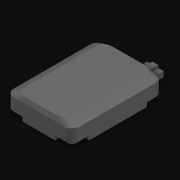
# Autodesk Inventor part: V5 Simple Brain
Saved by Autodesk Inventor 2025.2 (Build 292293000, 293)
## iProperties
Created: 2020-06-02
Part Number: V5 Simple Brain
Material: Generic
Document SubType Name: Modeling
Designer: yuany
Density: 1 g/cm^3
Appearance: Default
Author: yuany
Autodesk Inventor part; units mm, degrees
ref_plane "YZ Plane" through (0, 0, 0) normal (1, 0, 0) x (0, 1, 0)
ref_plane "XZ Plane" through (0, 0, 0) normal (0, 1, 0) x (-1, 0, 0)
ref_plane "XY Plane" through (0, 0, 0) normal (0, 0, 1) x (1, 0, 0)
sketch "Sketch1" plane through (0, 0, 0) normal (0, 1, 0) x (-1, 0, 0)
  line L0 (-49.911, 68.961) -> (49.911, 68.961)
  line L1 (49.911, 68.961) -> (49.911, -68.961)
  line L2 (49.911, -68.961) -> (-49.911, -68.961)
  line L3 (-49.911, -68.961) -> (-49.911, 68.961)
  point P0 (0, 0)
  dimension "d0" = 137.922
  dimension "d1" = 99.822
  dimension "d66" = 49.911
  dimension "d67" = 68.961
  constraints: 8 end point, 2 parallel, 1 horizontal, 1 perpendicular
  measures "d0" distance of L0.end L1.end
  measures "d1" distance of L1.end L2.end
  measures "d66" distance from line of point (0, 0) L1
  measures "d67" distance from line of point (0, 0) L0
extrude "Extrusion1" add sketch "Sketch1" along normal mid plane 31.4706
chamfer "Chamfer2" distance 2.921 distance2 6.35 1 edges at (0, 15.7353, 68.961) measured on face at (0, 15.7353, 68.461)
chamfer "Chamfer3" distance 2.921 distance2 6.35 1 edges at (0, 15.7353, -68.961) measured on face at (0, 15.7353, -68.461)
chamfer "Chamfer4" distance 12.7 distance2 6.35 1 edges at (49.911, 15.7353, 0) measured on face at (49.411, 15.7353, 0)
chamfer "Chamfer5" distance 12.7 distance2 6.35 1 edges at (-49.911, 15.7353, 0) measured on face at (-49.411, 15.7353, 0)
fillet "Fillet5" radius 11.811 8 edges at (-49.911, -3.175, -68.961) (-49.911, -3.175, 68.961) (49.911, -3.175, -68.961) (-43.561, 12.5603, -67.5005) (-43.561, 12.5603, 67.5005) (43.561, 12.5603, 67.5005) (43.561, 12.5603, -67.5005) (49.911, -3.175, 68.961)
fillet "Fillet6" radius 6.35 7 edges at (-46.4516, -15.7353, 65.5016) (0, -15.7353, 68.961) (49.911, -15.7353, 0) (46.4516, -15.7353, -65.5016) (0, -15.7353, -68.961) (-46.4516, -15.7353, -65.5016) (-49.911, -15.7353, 0) inverted yes
sketch "Sketch4" plane through (-49.911, 9.3853, -57.15) normal (-1, 0, 0) x (0, 0, 1)
  line L0 (114.3, -25.1206) -> (0, -25.1206) projected
  line L1 (12.7, -16.8159) -> (101.6, -16.8159)
  line L2 (101.6, -16.8159) -> (101.6, -25.1206)
  line L3 (101.6, -25.1206) -> (12.7, -25.1206)
  line L4 (12.7, -25.1206) -> (12.7, -16.8159)
  line L5 (0, 0) -> (114.3, 0) projected
  point P0 (57.15, -9.3853)
  point P1 (12.7, -25.1206)
  point P2 (119.761, -25.1206)
  dimension "d34" = 88.9
  dimension "d35" = 12.7
  constraints: 8 end point, 2 parallel, 1 horizontal, 1 perpendicular, 1 point on line
  measures "d34" distance of L2.end L3.end
  measures "d35" distance from line of L5.start L4
extrude "Extrusion4" add sketch "Sketch4" against normal up to surface (99.822 mm away)
sketch "Sketch5" plane through (-33.3726, 9.3853, 68.961) normal (0, 0, 1) x (1, 0, 0)
  line L0 (7.9756, -14.607) -> (58.7756, -14.607)
  line L1 (58.7756, -14.607) -> (58.7756, -25.1206)
  line L2 (58.7756, -25.1206) -> (7.9756, -25.1206)
  line L3 (7.9756, -25.1206) -> (7.9756, -14.607)
  line L4 (0, 0) -> (66.7451, 0) projected
  point P0 (33.3726, -9.3853)
  dimension "d38" = 50.8
  dimension "d39" = 7.9756
  constraints: 8 end point, 2 parallel, 1 horizontal, 1 perpendicular
  measures "d38" distance of L1.end L2.end
  measures "d39" distance from line of L4.start L3
extrude "Extrusion5" add sketch "Sketch5" against normal up to surface (137.922 mm away)
fillet "Fillet7" radius 2.0066 8 edges at (25.403, -15.7353, 65.786) (46.736, -15.7353, 44.45) (-25.397, -15.7353, 65.786) (-46.736, -15.7353, 44.45) (-46.736, -15.7353, -44.45) (-25.397, -15.7353, -65.786) (46.736, -15.7353, -44.45) (25.403, -15.7353, -65.786)
fillet "Fillet8" radius 0.254 47 edges at (43.5812, -15.2289, -43.776) (46.1975, -10.5844, -44.45) (46.4516, -9.3853, -65.5016) (31.7515, -9.3853, -68.961) (49.911, -9.3853, -50.8) (49.911, -15.1476, -43.8623) (49.911, -15.7353, 0) (49.911, -15.1476, 43.8623) (49.911, -11.557, 44.45) (49.911, -11.557, -44.45) (24.729, -15.2289, -62.6312) (25.403, -10.5844, -65.2475) (24.8153, -15.1476, -68.961) (0.003, -15.7353, -68.961) (-24.8092, -15.1476, -68.961) (-25.397, -11.557, -68.961) (25.403, -11.557, -68.961) (24.7268, -15.2309, 62.6311) (25.403, -10.5844, 65.2475) (49.911, -9.3853, 50.8) (31.7515, -9.3853, 68.961) (-31.7485, -9.3853, 68.961) (24.8153, -15.1476, 68.961) (0.003, -15.7353, 68.961) (-24.8092, -15.1476, 68.961) (-25.397, -11.557, 68.961) (25.403, -11.557, 68.961) (43.5812, -15.2289, 43.776) (46.1975, -10.5844, 44.45) (-43.5812, -15.2289, 43.776) (-46.1975, -10.5844, 44.45) (-46.4516, -9.3853, 65.5016) (-49.911, -9.3853, 50.8) (-24.723, -15.2289, 62.6312) (-25.397, -10.5844, 65.2475) (-49.911, -15.1476, 43.8623) (-49.911, -11.557, 44.45) (-49.911, -15.1476, -43.8623) (-49.911, -11.557, -44.45) (-49.911, -15.7353, 0) (-24.723, -15.2289, -62.6312) (-25.397, -10.5844, -65.2475) (-43.5812, -15.2289, -43.776) (-46.1975, -10.5844, -44.45) (-46.4516, -9.3853, -65.5016) (-31.7485, -9.3853, -68.961) (-49.911, -9.3853, -50.8)
sketch "Sketch6" plane through (0, -15.7353, 0) normal (0, -1, 0) x (1, 0, 0)
  circle A0 centre (19.053, 38.1) radius 1.7272
  line L0 (49.657, 42.4434) -> (49.657, -42.4434) projected
  line L1 (-23.3904, 68.707) -> (23.3964, 68.707) projected
  circle A1 centre (19.053, -38.1) radius 1.7272
  circle A2 centre (-19.047, 38.1) radius 1.7272
  circle A3 centre (-19.047, -38.1) radius 1.7272
  point P0 (0, 0)
  dimension "d44" = 3.4544
  dimension "d47" = 76.2
  dimension "d50" = 38.1
  dimension "d53" = 4.3434
  dimension "d54" = 4.3434
  constraints: 4 centre point, 1 horizontal, 1 vertical, 6 other
  measures "d44" diameter of A0
  measures "d47" distance of A0.centre A1.centre
  measures "d50" distance of A0.centre A2.centre
  measures "d53" vertical distance of A0.centre L0.start
  measures "d54" horizontal distance of A0.centre L1.end
extrude "Extrusion6" cut sketch "Sketch6" against normal blind 6.35
sketch "Sketch7" plane through (33.3726, 9.3853, -68.961) normal (0, 0, -1) x (-1, 0, 0)
  line L0 (-0.9809, -5.8547) -> (23.7079, -5.8547)
  line L1 (23.7079, -5.8547) -> (23.7079, -14.0843)
  line L2 (23.7079, -14.0843) -> (-0.9809, -14.0843)
  line L3 (-0.9809, -14.0843) -> (-0.9809, -5.8547)
  line L4 (6.9693, -5.8547) -> (15.8085, -5.8547)
  line L5 (15.8085, -5.8547) -> (15.8085, -1.9685)
  line L6 (15.8085, -1.9685) -> (6.9693, -1.9685)
  line L7 (6.9693, -1.9685) -> (6.9693, -5.8547)
  line L8 (-16.5384, 0) -> (-16.5384, -18.5215) projected
  line L9 (9.9761, -25.1206) -> (56.7629, -25.1206) projected
  point P0 (33.3726, -9.3853)
  point P1 (15.8085, -5.8547)
  dimension "d57" = 24.6888
  dimension "d58" = 8.2296
  dimension "d59" = 8.8392
  dimension "d60" = 3.8862
  dimension "d61" = 7.9502
  dimension "d62" = 15.5575
  dimension "d63" = 11.0363
  constraints: 16 end point, 4 parallel, 2 horizontal, 2 perpendicular, 1 point on line
  measures "d57" distance of L1.end L2.end
  measures "d58" distance of L0.end L1.end
  measures "d59" distance of L6.end L5.end
  measures "d60" distance of L5.end L4.end
  measures "d61" distance between parallel lines of L3 L7
  measures "d62" distance between parallel lines of L3 L8
  measures "d63" distance between parallel lines of L2 L9
extrude "Extrusion7" add sketch "Sketch7" along normal blind 15.875
equation "\"d66\" = 0.5 * d1"
equation "\"d67\" = 0.5 * d0"
body "Solid1"
